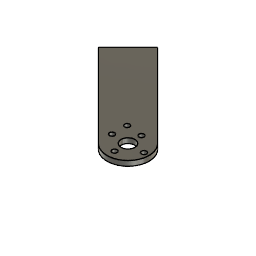
soporterbrushless (Autodesk Fusion 360 design; units mm, degrees)
Autodesk Fusion 360 part; units mm, degrees
sketch "Boceto1" plane through (0, 0, 0) normal (0, 0, 1) x (1, 0, 0)
  circle A0 centre (0, 0) radius 12.5
  circle A1 centre (0, 0) radius 4.1
  circle A2 centre (-9.5, 0) radius 1.5
  line L0 (0, 0) -> (0, 12.5)
  line L1 (0, 0) -> (-12.5, 0)
  circle A3 centre (9.5, 0) radius 1.5
  circle A4 centre (0, 8) radius 1.5
  circle A5 centre (0, -8) radius 1.5
  dimension "d1" = 25
  dimension "d2" = 8.2
  dimension "d3" = 3
  dimension "d4" = 9.5
  dimension "d5" = 3
  dimension "d6" = 8
  constraint coincident A0.centre A1.centre
  constraint horizontal A0.centre A2.centre
  constraint coincident A0 L0.end
  constraint vertical L0
  constraint coincident A0 L1.end
  constraint perpendicular L0 L1
  constraint symmetric A2 L0 A3
  constraint coincident L0 A4.centre
  constraint symmetric L1 A4 A5
  measures "d1" diameter of A0
  measures "d2" diameter of A1
  measures "d3" diameter of A2
  measures "d4" horizontal distance of A0.centre A2.centre
  measures "d5" diameter of A4
  measures "d6" distance of L1 A4.centre
extrude "Extruir1" add sketch "Boceto1" along normal blind 2 contours A0 A1 A2 L0 L1 A4 | A0 A1 A2 L0 L1 A4
sketch "Boceto2" plane through (0, 0, 2) normal (0, 0, 1) x (-1, 0, 0)
  circle A0 centre (9.5, 0) radius 1.5
  circle A1 centre (-9.5, 0) radius 1.5
  circle A2 centre (0, 8) radius 1.5
  circle A3 centre (0, 0) radius 4.1
  circle A4 centre (0, -8) radius 1.5
  circle A5 centre (0, 0) radius 12.5
  circle A6 centre (0, 0) radius 90
  dimension "d9" = 180
  constraint coincident A3.centre A5.centre
  measures "d9" diameter of A6
sketch "Boceto3" plane through (0, 0, 2) normal (0, 0, 1) x (-1, 0, 0)
  line L0 (8.4997, -8.4997) -> (49.4975, -49.4975)
  line L1 (-8.4997, -8.4997) -> (-8.8356, -8.8356)
  line L2 (-8.8356, -8.8356) -> (40.6619, -58.3331)
  line L3 (8.8356, 8.8356) -> (58.3331, -40.6619)
  line L4 (8.4997, 8.4997) -> (8.8356, 8.8356)
  line L5 (40.6619, -58.3331) -> (58.3331, -40.6619)
  arc A0 (-8.4997, -8.4997) -> (8.4997, 8.4997) centre (0, 0) ccw
  dimension "d10" = 70
  dimension "d11" = 70
  constraint perpendicular L0 L1
  constraint perpendicular L1 L2
  constraint symmetric L0 L1.end L3.start
  constraint symmetric L0 L2.end L3.end
  constraint coincident A0 L0.start
  measures "d10" distance of A0.centre L0.end
  measures "d11" distance of L1.end L2.end
extrude "Extruir2" add sketch "Boceto3" against normal blind 2
sketch "Boceto4" plane through (-49.4975, 49.4975, 0) normal (-0.707107, 0.707107, 0) x (-0.707107, -0.707107, 0)
  line L0 (12.4955, 2) -> (-12.4955, 2)
  line L1 (-12.4955, 2) -> (-12.4955, 0)
  line L2 (-12.4955, 0) -> (12.4955, 0)
  line L3 (12.4955, 0) -> (12.4955, 2)
  line L4 (12.4955, 2) -> (-12.4986, 2)
  line L5 (-12.4986, 2) -> (-12.4986, -27)
  line L6 (-12.4986, -27) -> (12.4955, -27)
  line L7 (12.4955, -27) -> (12.4955, 2)
  constraint horizontal L4
  constraint vertical L5
  constraint horizontal L6
  constraint vertical L7
  constraint coincident L0.start L3.end
extrude "Extruir3" add sketch "Boceto4" against normal blind 3 contours L1 L2 L4 L5 L6 L7
sketch "Boceto5" plane through (-47.3762, 47.3762, 0) normal (0.707107, -0.707107, 0) x (0.707107, 0.707107, 0)
  line L0 (12.4986, -27) -> (12.4986, 2)
  line L1 (12.4955, 0) -> (-12.4955, 0)
  line L2 (-12.4955, 0) -> (-12.4955, -27)
  line L3 (-12.4955, -27) -> (12.4986, -27)
  circle A0 centre (-8.9991, -3.0002) radius 1.5
  line L4 (0, 0) -> (0.0016, -27)
  line L5 (0.0008, -13.5) -> (-12.4955, -13.5)
  circle A1 centre (-8.9991, -23.9998) radius 1.5
  circle A2 centre (9.0018, -23.9988) radius 1.5
  circle A3 centre (8.9994, -2.9991) radius 1.5
  line L6 (0, 0) -> (0.0016, -27)
  line L7 (12.4986, 2) -> (12.4955, 2)
  line L8 (12.4955, 2) -> (12.4955, 0)
  dimension "d16" = 3
  constraint coincident L4.start L6.start
  constraint midpoint L3 L4.end
  constraint midpoint L4 L5.start
  constraint midpoint L2 L5.end
  constraint symmetric A0 L5 A1
  constraint symmetric A0 L4 A3
  constraint symmetric L6.start L4 origin
  constraint symmetric L6.end L4 L4.end
  constraint symmetric L4 A1 A2
  measures "d16" diameter of A0
extrude "Extruir5" add sketch "Boceto3" sketch "Boceto2" along normal blind 1 of sketch 2 contours A5
sketch "Boceto6" plane through (0, 0, 0) normal (0, 0, -1) x (1, 0, 0)
  circle A0 centre (-9.5, 0) radius 1.5
  circle A1 centre (9.5, 0) radius 1.5
  circle A2 centre (0, 8) radius 1.5
  circle A3 centre (0, 0) radius 4.1
  circle A4 centre (0, -8) radius 1.5
  line L0 (-56.2118, -38.5405) -> (-38.5405, -56.2118)
  line L1 (-38.5405, -56.2118) -> (8.5973, -9.0739)
  arc A5 (8.5973, -9.0739) -> (-9.0739, 8.5973) centre (0, 0) ccw
  line L2 (-9.0739, 8.5973) -> (-56.2118, -38.5405)
  circle A6 centre (-9.4144, -8.9402) radius 1.5
  dimension "d25" = 3
  measures "d25" diameter of A6
sketch "Boceto7" plane through (-8.8356, -8.8356, 0) normal (-0.707107, -0.707107, 0) x (0.707107, -0.707107, 0)
  line L0 (-0.337, 0) -> (-0.337, 3)
  line L1 (-0.337, 3) -> (-70, 3)
  line L2 (-70, 3) -> (-70, -27)
  line L3 (-70, -27) -> (-67, -27)
  line L4 (-67, -27) -> (-67, 0)
  line L5 (-67, 0) -> (-0.337, 0)
  line L6 (-67, -27) -> (-16, 0)
  line L7 (-67, -27) -> (-67, 0)
  line L8 (-67, 0) -> (-16, 0)
  constraint coincident L3.end L4.start
  constraint coincident L5 L6.end
  constraint coincident L4.end L5.start
extrude "Extruir7" add sketch "Boceto7" against normal blind 16 contours L4 L5 L6 L7 L8
extrude "Extruir8" cut sketch "Boceto7" against normal blind 9 contours L4 L5 L6 L7 L8
extrude "Extruir6" cut sketch "Boceto6" along normal mid plane 16 contours A6
sketch "Boceto8" plane through (-47.3762, 47.3762, 0) normal (0.707107, -0.707107, 0) x (0.707107, 0.707107, 0)
  line L0 (-12.4955, 0) -> (-12.4955, -27)
  line L1 (-12.4955, -27) -> (-3.4955, -27)
  line L2 (-3.4955, -27) -> (-3.4955, 0)
  line L3 (-3.4955, 0) -> (-12.4955, 0)
  line L4 (0, 0) -> (0, -27)
  line L5 (0, -13.5) -> (-3.4955, -13.5)
  line L6 (-3.4955, -13.5) -> (-12.4955, -13.5)
  circle A0 centre (-7.9955, -13.5) radius 1.6
  line L7 (0, -13.5) -> (3.5, -13.5)
  line L8 (3.5, -13.5) -> (12.5, -13.5)
  circle A1 centre (8, -13.5) radius 1.6
  dimension "d32" = 3.2
  dimension "d33" = 3.2
  constraint coincident L4.start origin
  constraint perpendicular L3 L4
  constraint midpoint L4 L5.start
  constraint midpoint L2 L5.end
  constraint midpoint L0 L6.end
  constraint midpoint L6 A0.centre
  constraint perpendicular L4 L7
  constraint perpendicular L4 L8
  constraint midpoint L8 A1.centre
  measures "d32" diameter of A0
  measures "d33" diameter of A1
extrude "Extruir9" cut sketch "Boceto8" against normal blind 9 contours L6 A0 | L6 A0 | L8 A1 | L8 A1
